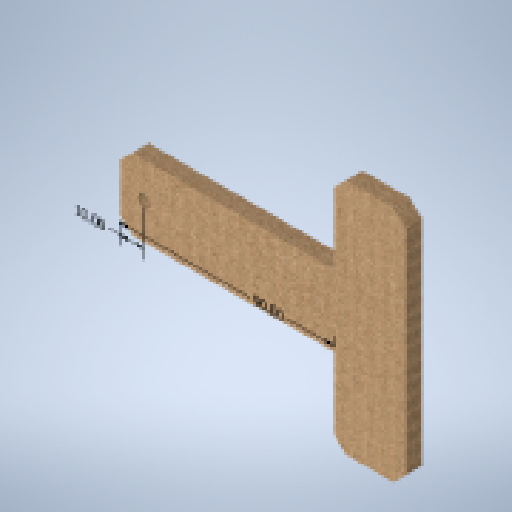
# Autodesk Inventor part: PistonV2
Saved by Autodesk Inventor 2023.1 (Build 271208000, 208)
## iProperties
Created: 2022-10-30
Part Number: PistonV2
Material: MDF Medium Density Fiberboard
Document SubType Name: Modeling
Designer: Daniel Peña
Density: 0.8 g/cm^3
Appearance: Cardboard - Corrugated
Author: Daniel Peña
Autodesk Inventor part; units mm, degrees
ref_plane "YZ Plane" through (0, 0, 0) normal (1, 0, 0) x (0, 1, 0)
ref_plane "XZ Plane" through (0, 0, 0) normal (0, 1, 0) x (-1, 0, 0)
ref_plane "XY Plane" through (0, 0, 0) normal (0, 0, 1) x (1, 0, 0)
sketch "Sketch1" plane through (0, 0, 0) normal (0, 0, 1) x (1, 0, 0)
  line L0 (120.5719, -15.0856) -> (100.5719, -15.0856)
  line L1 (100.5719, -115.0856) -> (120.5719, -115.0856)
  line L2 (125.5719, -110.0856) -> (125.5719, -20.0856)
  line L3 (95.5719, -50.0856) -> (10.5719, -50.0856)
  line L4 (5.5719, -55.0856) -> (5.5719, -75.0856)
  line L5 (10.5719, -80.0856) -> (95.5719, -80.0856)
  line L6 (95.5719, -20.0856) -> (95.5719, -50.0856)
  line L7 (95.5719, -80.0856) -> (95.5719, -110.0856)
  line L8 (125.5719, -65.0856) -> (5.5719, -65.0856) construction
  line L9 (125.5719, -20.0856) -> (120.5719, -15.0856)
  line L10 (100.5719, -15.0856) -> (95.5719, -20.0856)
  line L11 (120.5719, -115.0856) -> (125.5719, -110.0856)
  line L12 (100.5719, -115.0856) -> (95.5719, -110.0856)
  line L13 (10.5719, -80.0856) -> (5.5719, -75.0856)
  line L14 (5.5719, -55.0856) -> (10.5719, -50.0856)
  point P0 (0, 0)
  point P1 (125.5719, -15.0856)
  point P2 (95.5719, -115.0856)
  point P3 (95.5719, -15.0856)
  point P4 (125.5719, -115.0856)
  point P5 (5.5719, -80.0856)
  point P6 (5.5719, -50.0856)
  point P7 (15.5719, -65.0856)
  dimension "d0" = 30
  dimension "d3" = 30
  dimension "d4" = 100
  dimension "d5" = 5
  dimension "d6" = 5
  dimension "d7" = 5
  dimension "d8" = 5
  dimension "d9" = 5
  dimension "d10" = 5
  dimension "d11" = 5
  dimension "d12" = 5
  dimension "d13" = 5
  dimension "d14" = 5
  dimension "d15" = 5
  dimension "d16" = 5
  dimension "d33" = 10
  dimension "d37" = 90
  constraints: 30 end point, 13 point on line, 4 parallel, 4 perpendicular, 2 horizontal, 2 midpoint, 1 collinear, 1 other
  measures "d0" distance of point (125.572, -115.086) point (95.572, -115.086)
  measures "d3" distance of point (5.572, -80.086) point (5.572, -50.086)
  measures "d4" distance between parallel lines of L1 L0
  measures "d5" distance of L2.end point (125.572, -15.086)
  measures "d6" distance of L0.start point (125.572, -15.086)
  measures "d7" distance of L0.end point (95.572, -15.086)
  measures "d8" distance of L6.start point (95.572, -15.086)
  measures "d9" distance of L1.end point (125.572, -115.086)
  measures "d10" distance of L2.start point (125.572, -115.086)
  measures "d11" distance of L1.start point (95.572, -115.086)
  measures "d12" distance of L7.end point (95.572, -115.086)
  measures "d13" distance of L5.start point (5.572, -80.086)
  measures "d14" distance of L4.end point (5.572, -80.086)
  measures "d15" distance of L4.start point (5.572, -50.086)
  measures "d16" distance of L3.end point (5.572, -50.086)
  measures "d33" distance from line of L4 point (15.572, -65.086)
  measures "d37" distance between parallel lines of L7 L4
extrude "Extrusion1" add sketch "Sketch1" along normal blind 7
sketch "Sketch2" plane through (0, 0, 7) normal (0, 0, 1) x (1, 0, 0)
  line L0 (5.5719, -55.0856) -> (5.5719, -75.0856) projected
  line L1 (10.5719, -80.0856) -> (95.5719, -80.0856) projected
  point P0 (0, 0)
  point P1 (15.5719, -65.0856)
  dimension "d19" = 10
  dimension "d27" = 15
  measures "d19" distance from line of L0 point (15.572, -65.086)
  measures "d27" distance from line of L1 point (15.572, -65.086)
hole "Hole1" at (15.5719, -65.0856, 7) direction (0, 0, -1) diameter 5 end through all
equation "\"d6\" = d5"
equation "\"d7\" = d5"
equation "\"d8\" = d7"
equation "\"d9\" = d5"
equation "\"d10\" = d9"
equation "\"d11\" = d5"
equation "\"d12\" = d11"
equation "\"d13\" = d5"
equation "\"d14\" = d13"
equation "\"d15\" = d5"
equation "\"d16\" = d15"
body "Solid1"
